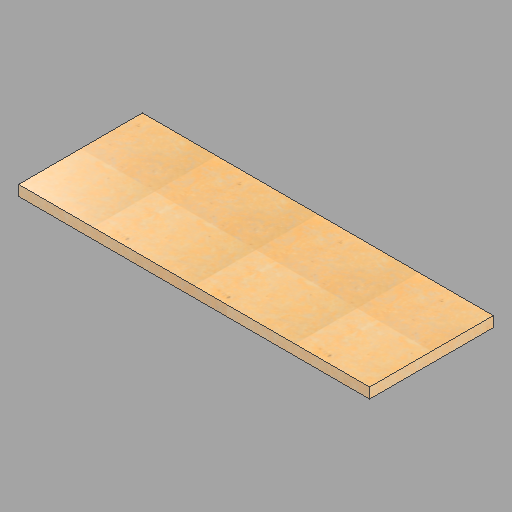
# Autodesk Inventor part: 15 - lid - 4
Saved by Autodesk Inventor 2023 (Build 270158030, 158C)
## iProperties
RuleStatus: InUse
Created: 2022-03-21
Part Number: 15 - lid - 4
Material: Granite, Cut, Polished
Document SubType Name: Modeling
Designer: awelt
Mass: 477598 g
Surface Area: 51716 cm^2
Volume: 176888 cm^3
Density: 2.7 g/cm^3
Appearance: Amber Select
AfterDocSave0: Convert in3 volume to ft3
in3 to ft3: 6.25
TEST: 6.247
Author: awelt
Autodesk Inventor part; units mm, degrees
ref_plane "YZ Plane" through (0, 0, 0) normal (1, 0, 0) x (0, 1, 0)
ref_plane "XZ Plane" through (0, 0, 0) normal (0, 1, 0) x (-1, 0, 0)
ref_plane "XY Plane" through (0, 0, 0) normal (0, 0, 1) x (1, 0, 0)
sketch "Sketch1" plane through (0, 0, 0) normal (0, 1, 0) x (-1, 0, 0)
  line L0 (1282.7, -452.4375) -> (-1282.7, -452.4375)
  line L1 (-1282.7, -452.4375) -> (-1282.7, 452.4375)
  line L2 (-1282.7, 452.4375) -> (1282.7, 452.4375)
  line L3 (1282.7, 452.4375) -> (1282.7, -452.4375)
  line L4 (1282.7, -452.4375) -> (-1282.7, 452.4375) construction
  line L5 (-1282.7, -452.4375) -> (1282.7, 452.4375) construction
  point P0 (0, 0)
  dimension "d0" = 2565.4
  dimension "d1" = 904.875
  constraints: 12 end point, 2 midpoint, 2 parallel, 1 horizontal, 1 perpendicular
  measures "d0" distance of L1.end L2.end
  measures "d1" distance of L0.end L1.end
extrude "Extrusion1" add sketch "Sketch1" along normal blind 76.2
body "Solid1"
